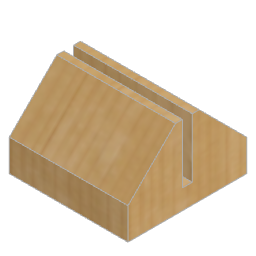
_Plank Barrier Tower.620c9861-89cf-472f-92b7-07eff5aa2384 (Autodesk Fusion 360 design; units mm, degrees)
Autodesk Fusion 360 part; units mm, degrees
sketch "Sketch1" plane through (0, 0, 0) normal (0, 0, 1) x (1, 0, 0)
  line L0 (0, 0) -> (-38.1, 0)
  line L1 (-38.1, 0) -> (-38.1, 38.1)
  line L2 (-38.1, 38.1) -> (0, 38.1)
  line L3 (0, 38.1) -> (0, 0)
  dimension "d1" = 38.1
  dimension "d2" = 38.1
  constraint horizontal L0
  constraint vertical L1
  constraint horizontal L2
  constraint vertical L3
  constraint coincident L0.start L3.end
  measures "d1" distance of L0.start L0.end
  measures "d2" distance of L0.start L2.end
extrude "Extrude1" add sketch "Sketch1" along normal blind 25.4
chamfer "Chamfer1" distance 15.24 angle 45 2 edges at (-19.05, 0, 25.4) (-19.05, 38.1, 25.4)
sketch "Sketch2" plane through (0, 0, 25.4) normal (0, 0, 1) x (-1, 0, 0)
  line L0 (0, -22.86) -> (38.1, -22.86)
  line L1 (38.1, -22.86) -> (38.1, -15.24)
  line L2 (38.1, -15.24) -> (0, -15.24)
  line L3 (0, -15.24) -> (0, -22.86)
  line L4 (38.1, -19.05) -> (0, -19.05)
  line L5 (0, -19.05) -> (0, -20.6375)
  line L6 (0, -20.6375) -> (38.1, -20.6375)
  line L7 (38.1, -20.6375) -> (38.1, -19.05)
  line L8 (38.1, -19.05) -> (0, -19.05)
  line L9 (0, -19.05) -> (0, -17.4625)
  line L10 (0, -17.4625) -> (38.1, -17.4625)
  line L11 (38.1, -17.4625) -> (38.1, -19.05)
  dimension "d6" = 1.5875
  dimension "d7" = 1.5875
  constraint horizontal L4
  constraint vertical L5
  constraint horizontal L6
  constraint vertical L7
  constraint midpoint L1 L4.start
  constraint horizontal L8
  constraint vertical L9
  constraint horizontal L10
  constraint vertical L11
  measures "d6" distance of L4.start L6.end
  measures "d7" distance of L4.start L10.end
extrude "Extrude2" cut sketch "Sketch2" against normal blind 19.05 contours L1 L3 L4 L5 L6 L7 L8 | L1 L3 L4 L8 L9 L10 L11
sketch "Sketch3" plane through (0, 0, 0) normal (0, 0, -1) x (1, 0, 0)
  line L0 (-38.1, -38.1) -> (0, -38.1)
  line L1 (0, -38.1) -> (0, 0)
  line L2 (0, 0) -> (-38.1, 0)
  line L3 (-38.1, 0) -> (-38.1, -38.1)
  circle A0 centre (-19.05, -19.05) radius 15.875
  dimension "d10" = 31.75
  measures "d10" diameter of A0
extrude "Extrude3" cut sketch "Sketch3" against normal blind 3.175 contours A0
